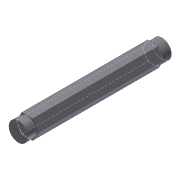
# Autodesk Inventor part: AM shifter new input shaft
Saved by Autodesk Inventor 2011 SP1 (Build 150282100, 282)
## iProperties
Created: 2011-07-15
Part Number: AM shifter new input shaft
Material: Steel
Document SubType Name: Modeling
Designer: Dan Niemitalo
Mass: 43.3515 g
Surface Area: 24.8706 cm^2
Volume: 5.52248 cm^3
Density: 7.85 g/cm^3
Author: Dan Niemitalo
Autodesk Inventor part; units mm, degrees
ref_plane "YZ Plane" through (0, 0, 0) normal (1, 0, 0) x (0, 1, 0)
ref_plane "XZ Plane" through (0, 0, 0) normal (0, 1, 0) x (-1, 0, 0)
ref_plane "XY Plane" through (0, 0, 0) normal (0, 0, 1) x (1, 0, 0)
sketch "Sketch1" plane through (0, 0, 0) normal (0, 0, 1) x (1, 0, 0)
  line L0 (-2.735, 4.7371) -> (2.735, 4.7371)
  line L1 (2.735, 4.7371) -> (5.4699, 0)
  line L2 (5.4699, 0) -> (2.735, -4.7371)
  line L3 (2.735, -4.7371) -> (-2.735, -4.7371)
  line L4 (-2.735, -4.7371) -> (-5.4699, 0)
  line L5 (-5.4699, 0) -> (-2.735, 4.7371)
  point P0 (0, 0)
  point P1 (0, 0)
  dimension "d0" = 9.4742
  constraints: 12 end point, 1 coincident, 1 horizontal, 13 other
  measures "d0" distance between parallel lines of L3 L0
extrude "Extrusion1" add sketch "Sketch1" along normal mid plane 62.992
sketch "Sketch2" plane through (0, 0, 31.496) normal (0, 0, 1) x (1, 0, 0)
  circle A0 centre (0, 0) radius 4.7371
  dimension "d3" = 9.4742
  constraints: 1 centre point, 1 coincident
  measures "d3" diameter of A0
extrude "Extrusion2" add sketch "Sketch2" along normal blind 4.445
sketch "Sketch3" plane through (0, 0, -31.496) normal (0, 0, -1) x (-1, 0, 0)
  circle A0 centre (0, 0) radius 4.7371
  dimension "d6" = 9.4742
  constraints: 1 centre point, 1 coincident
  measures "d6" diameter of A0
extrude "Extrusion3" add sketch "Sketch3" along normal blind 4.445
body "Solid1"
